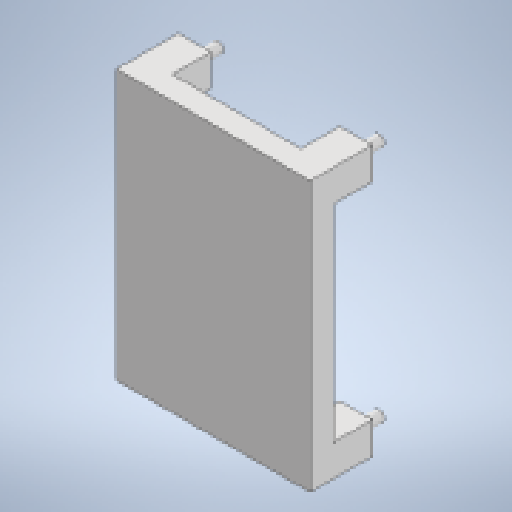
# Autodesk Inventor part: head_box
Saved by Autodesk Inventor 2024 (Build 280153000, 153)
## iProperties
Created: 2024-09-18
Part Number: head_box
Material: 일반
Document SubType Name: Modeling
Designer: Eungang
Density: 1 g/cm^3
Appearance: 기본값
Author: Eungang
Autodesk Inventor part; units mm, degrees
ref_plane "YZ Plane" through (0, 0, 0) normal (1, 0, 0) x (0, 1, 0)
ref_plane "XZ Plane" through (0, 0, 0) normal (0, 1, 0) x (-1, 0, 0)
ref_plane "XY Plane" through (0, 0, 0) normal (0, 0, 1) x (1, 0, 0)
sketch "스케치1" plane through (0, 0, 0) normal (0, 0, 1) x (1, 0, 0)
  circle A0 centre (20.8, -30.8) radius 1.6
  circle A1 centre (20.8, 30.8) radius 1.6
  circle A2 centre (-20.8, -30.8) radius 1.6
  circle A3 centre (-20.8, 30.8) radius 1.6
  line L0 (25, 35) -> (25, -35)
  line L1 (-25, 35) -> (25, 35)
  line L2 (-25, -35) -> (-25, 35)
  line L3 (25, -35) -> (-25, -35)
  line L4 (3.4609, -14.6309) -> (3.4609, -15.4416)
  line L5 (3.4609, -15.4416) -> (-1.9174, -15.4416)
  line L6 (-1.9174, -15.4416) -> (-1.9174, -17.4882)
  line L7 (-1.9174, -17.4882) -> (-2.6391, -17.4882)
  line L8 (-2.6391, -17.4882) -> (-2.6391, -12.5844)
  line L9 (-2.6391, -12.5844) -> (-1.9174, -12.5844)
  line L10 (-1.9174, -12.5844) -> (-1.9174, -14.6309)
  line L11 (-1.9174, -14.6309) -> (3.4609, -14.6309)
  spline S0 degree 3 poles (3.5894, -6.7069) (3.5894, -7.2061) (3.5079, -7.4974) (3.4054, -7.7829) (3.3472, -7.9038) (3.2038, -8.1322) (3.1203, -8.2371) (3.0259, -8.3332) knots 0 0 0 0 0.384557 0.384557 0.692405 0.692405 1 1 1 1
  spline S1 degree 3 poles (3.0259, -8.3332) (2.8735, -8.4928) (2.696, -8.6163) (2.4131, -8.7398) (2.2257, -8.8143) (1.6618, -8.9024) (1.4109, -8.9165) (1.1672, -8.9165) knots 0 0 0 0 0.589252 0.589252 0.824533 0.824533 1 1 1 1
  line L12 (1.1672, -8.9165) -> (-2.6391, -8.9165)
  line L13 (-2.6391, -8.9165) -> (-2.6391, -8.1058)
  line L14 (-2.6391, -8.1058) -> (1.187, -8.1058)
  spline S2 degree 3 poles (1.187, -8.1058) (1.576, -8.1058) (1.7854, -8.0698) (2.0673, -8.0159) (2.2402, -7.948) (2.3981, -7.8438) knots 0 0 0 0 0.340954 0.340954 1 1 1 1
  spline S3 degree 3 poles (2.3981, -7.8438) (2.5057, -7.7728) (2.5951, -7.6834) (2.7648, -7.4325) (2.8129, -7.284) (2.8802, -7.0309) (2.8973, -6.8687) (2.8973, -6.7069) knots 0 0 0 0 0.220643 0.220643 0.518387 0.518387 1 1 1 1
  spline S4 degree 3 poles (2.8973, -6.7069) (2.8973, -6.4866) (2.8694, -6.2573) (2.7554, -5.9796) (2.7065, -5.8804) (2.5606, -5.7003) (2.4845, -5.6319) (2.3981, -5.5749) knots 0 0 0 0 0.605349 0.605349 0.823714 0.823714 1 1 1 1
  spline S5 degree 3 poles (2.3981, -5.5749) (2.2456, -5.4743) (2.0787, -5.4078) (1.787, -5.3484) (1.5677, -5.3129) (1.1672, -5.3129) knots 0 0 0 0 0.613521 0.613521 1 1 1 1
  line L15 (1.1672, -5.3129) -> (-2.6391, -5.3129)
  line L16 (-2.6391, -5.3129) -> (-2.6391, -4.5022)
  line L17 (-2.6391, -4.5022) -> (1.1672, -4.5022)
  spline S6 degree 3 poles (1.1672, -4.5022) (1.7467, -4.5022) (2.0771, -4.578) (2.4094, -4.6758) (2.5476, -4.7346) (2.8054, -4.8878) (2.9214, -4.9794) (3.0259, -5.0855) knots 0 0 0 0 0.39454 0.39454 0.699346 0.699346 1 1 1 1
  spline S7 degree 3 poles (3.0259, -5.0855) (3.188, -5.2476) (3.3119, -5.4359) (3.468, -5.8026) (3.513, -5.9645) (3.576, -6.3201) (3.5894, -6.5148) (3.5894, -6.7069) knots 0 0 0 0 0.387918 0.387918 0.674422 0.674422 1 1 1 1
  line L18 (3.4609, 6.6696) -> (2.838, 6.6696)
  line L19 (2.838, 6.6696) -> (2.838, 7.4457)
  line L20 (2.838, 7.4457) -> (-2.0163, 7.4457)
  line L21 (-2.0163, 7.4457) -> (-2.0163, 6.6696)
  line L22 (-2.0163, 6.6696) -> (-2.6391, 6.6696)
  line L23 (-2.6391, 6.6696) -> (-2.6391, 9.0325)
  line L24 (-2.6391, 9.0325) -> (-2.0163, 9.0325)
  line L25 (-2.0163, 9.0325) -> (-2.0163, 8.2564)
  line L26 (-2.0163, 8.2564) -> (2.838, 8.2564)
  line L27 (2.838, 8.2564) -> (2.838, 9.0325)
  line L28 (2.838, 9.0325) -> (3.4609, 9.0325)
  line L29 (3.4609, 9.0325) -> (3.4609, 6.6696)
  spline S8 degree 3 poles (3.5696, 11.4498) (3.5696, 11.0968) (3.5385, 10.9252) (3.4927, 10.6907) (3.4451, 10.5225) (3.3917, 10.3623) knots 0 0 0 0 0.292547 0.292547 1 1 1 1
  spline S9 degree 3 poles (3.3917, 10.3623) (3.3122, 10.1089) (3.2476, 9.9765) (3.1649, 9.8065) (3.1044, 9.6784) (3.0456, 9.5516) knots 0 0 0 0 0.260501 0.260501 1 1 1 1
  line L30 (3.0456, 9.5516) -> (2.0767, 9.5516)
  line L31 (2.0767, 9.5516) -> (2.0767, 9.6109)
  spline S10 degree 3 poles (2.0767, 9.6109) (2.1724, 9.7066) (2.276, 9.8355) (2.4013, 9.9909) (2.4887, 10.1245) (2.5661, 10.2584) knots 0 0 0 0 0.224538 0.224538 1 1 1 1
  spline S11 degree 3 poles (2.5661, 10.2584) (2.6936, 10.4889) (2.7578, 10.7089) (2.8422, 11.001) (2.8677, 11.2201) (2.8677, 11.4399) knots 0 0 0 0 0.277128 0.277128 1 1 1 1
  spline S12 degree 3 poles (2.8677, 11.4399) (2.8677, 11.6791) (2.8234, 11.9096) (2.6905, 12.2276) (2.6304, 12.347) (2.4562, 12.5833) (2.363, 12.6815) (2.2596, 12.7696) knots 0 0 0 0 0.549193 0.549193 0.79146 0.79146 1 1 1 1
  spline S13 degree 3 poles (2.2596, 12.7696) (2.0598, 12.9378) (1.8287, 13.0612) (1.3654, 13.2321) (1.0093, 13.3332) (0.4158, 13.3332) knots 0 0 0 0 0.528777 0.528777 1 1 1 1
  spline S14 degree 3 poles (0.4158, 13.3332) (-0.1058, 13.3332) (-0.4504, 13.2487) (-0.927, 13.104) (-1.2002, 12.9774) (-1.428, 12.7894) knots 0 0 0 0 0.407318 0.407318 1 1 1 1
  spline S15 degree 3 poles (-1.428, 12.7894) (-1.6106, 12.6333) (-1.7595, 12.4499) (-1.9192, 12.1338) (-1.9723, 12.0047) (-2.0407, 11.7153) (-2.0558, 11.5784) (-2.0558, 11.4399) knots 0 0 0 0 0.529795 0.529795 0.78096 0.78096 1 1 1 1
  spline S16 degree 3 poles (-2.0558, 11.4399) (-2.0558, 11.0983) (-1.9995, 10.8945) (-1.922, 10.6336) (-1.853, 10.4636) (-1.7642, 10.3029) knots 0 0 0 0 0.325292 0.325292 1 1 1 1
  spline S17 degree 3 poles (-1.7642, 10.3029) (-1.6346, 10.0678) (-1.5778, 9.9965) (-1.419, 9.8036) (-1.3331, 9.7017) (-1.255, 9.6158) knots 0 0 0 0 0.538227 0.538227 1 1 1 1
  line L32 (-1.255, 9.6158) -> (-1.255, 9.5516)
  line L33 (-1.255, 9.5516) -> (-2.2338, 9.5516)
  spline S18 degree 3 poles (-2.2338, 9.5516) (-2.3342, 9.7386) (-2.4001, 9.8833) (-2.4926, 10.0908) (-2.5452, 10.2254) (-2.5897, 10.3623) knots 0 0 0 0 0.366727 0.366727 1 1 1 1
  spline S19 degree 3 poles (-2.5897, 10.3623) (-2.6578, 10.586) (-2.6908, 10.783) (-2.7347, 11.0489) (-2.7479, 11.2426) (-2.7479, 11.4349) knots 0 0 0 0 0.286175 0.286175 1 1 1 1
  spline S20 degree 3 poles (-2.7479, 11.4349) (-2.7479, 11.8102) (-2.6884, 12.1794) (-2.4851, 12.6671) (-2.4001, 12.8345) (-2.1695, 13.1574) (-2.0458, 13.2939) (-1.9075, 13.4172) knots 0 0 0 0 0.566594 0.566594 0.797666 0.797666 1 1 1 1
  spline S21 degree 3 poles (-1.9075, 13.4172) (-1.6331, 13.6594) (-1.3194, 13.8381) (-0.7236, 14.0548) (-0.2884, 14.1785) (0.4158, 14.1785) knots 0 0 0 0 0.577352 0.577352 1 1 1 1
  spline S22 degree 3 poles (0.4158, 14.1785) (1.1016, 14.1785) (1.5387, 14.0598) (1.9684, 13.9147) (2.1514, 13.8354) (2.4841, 13.645) (2.6333, 13.5376) (2.7688, 13.4123) knots 0 0 0 0 0.205724 0.205724 0.366116 0.366116 0.515054 0.515054 0.515054 0.515054
  spline S23 degree 3 poles (2.7688, 13.4123) (3.001, 13.2001) (3.1844, 12.9521) (3.4019, 12.4833) (3.465, 12.2871) (3.55, 11.8776) (3.5696, 11.6642) (3.5696, 11.4498) knots 0 0 0 0 0.431078 0.431078 0.708336 0.708336 1 1 1 1
  line L34 (3.4609, 0.9453) -> (0.8063, 3.1154)
  spline S24 degree 3 poles (0.8063, 3.1154) (0.7091, 2.8546) (0.5712, 2.6157) (0.2499, 2.2703) (0.0734, 2.1207) (-0.2854, 1.9573) (-0.4142, 1.9172) (-0.6904, 1.8622) (-0.8369, 1.8499) (-0.9831, 1.8499) knots 0 0 0 0 0.408273 0.408273 0.691747 0.691747 0.83987 0.83987 1 1 1 1
  spline S25 degree 3 poles (-0.9831, 1.8499) (-1.2, 1.8499) (-1.421, 1.8784) (-1.7689, 2.0145) (-1.898, 2.0959) (-2.134, 2.2962) (-2.234, 2.4122) (-2.3178, 2.542) knots 0 0 0 0 0.409869 0.409869 0.705358 0.705358 1 1 1 1
  spline S26 degree 3 poles (-2.3178, 2.542) (-2.4457, 2.7399) (-2.5352, 2.9539) (-2.6309, 3.4845) (-2.6391, 3.7907) (-2.6391, 4.0942) knots 0 0 0 0 0.436998 0.436998 1 1 1 1
  line L35 (-2.6391, 4.0942) -> (-2.6391, 5.6661)
  line L36 (-2.6391, 5.6661) -> (3.4609, 5.6661)
  line L37 (3.4609, 5.6661) -> (3.4609, 4.8554)
  line L38 (3.4609, 4.8554) -> (1.0337, 4.8554)
  line L39 (1.0337, 4.8554) -> (1.0337, 3.9261)
  line L40 (1.0337, 3.9261) -> (3.4609, 1.9982)
  line L41 (3.4609, 1.9982) -> (3.4609, 0.9453)
  spline S27 degree 3 poles (3.5696, -1.9218) (3.5696, -2.2748) (3.5385, -2.4464) (3.4927, -2.6809) (3.4451, -2.849) (3.3917, -3.0093) knots 0 0 0 0 0.292547 0.292547 1 1 1 1
  spline S28 degree 3 poles (3.3917, -3.0093) (3.3122, -3.2627) (3.2476, -3.3951) (3.1649, -3.5651) (3.1044, -3.6932) (3.0456, -3.82) knots 0 0 0 0 0.260501 0.260501 1 1 1 1
  line L42 (3.0456, -3.82) -> (2.0767, -3.82)
  line L43 (2.0767, -3.82) -> (2.0767, -3.7607)
  spline S29 degree 3 poles (2.0767, -3.7607) (2.1724, -3.665) (2.276, -3.5361) (2.4013, -3.3806) (2.4887, -3.2471) (2.5661, -3.1131) knots 0 0 0 0 0.224538 0.224538 1 1 1 1
  spline S30 degree 3 poles (2.5661, -3.1131) (2.6936, -2.8826) (2.7578, -2.6627) (2.8422, -2.3706) (2.8677, -2.1514) (2.8677, -1.9317) knots 0 0 0 0 0.277128 0.277128 1 1 1 1
  spline S31 degree 3 poles (2.8677, -1.9317) (2.8677, -1.6925) (2.8234, -1.462) (2.6905, -1.144) (2.6304, -1.0246) (2.4562, -0.7882) (2.363, -0.6901) (2.2596, -0.6019) knots 0 0 0 0 0.549193 0.549193 0.79146 0.79146 1 1 1 1
  spline S32 degree 3 poles (2.2596, -0.6019) (2.0598, -0.4338) (1.8287, -0.3103) (1.3654, -0.1394) (1.0093, -0.0384) (0.4158, -0.0384) knots 0 0 0 0 0.528777 0.528777 1 1 1 1
  spline S33 degree 3 poles (0.4158, -0.0384) (-0.1058, -0.0384) (-0.4504, -0.1228) (-0.927, -0.2675) (-1.2002, -0.3941) (-1.428, -0.5822) knots 0 0 0 0 0.407318 0.407318 1 1 1 1
  spline S34 degree 3 poles (-1.428, -0.5822) (-1.6106, -0.7383) (-1.7595, -0.9217) (-1.9192, -1.2377) (-1.9723, -1.3669) (-2.0407, -1.6563) (-2.0558, -1.7931) (-2.0558, -1.9317) knots 0 0 0 0 0.529795 0.529795 0.78096 0.78096 1 1 1 1
  spline S35 degree 3 poles (-2.0558, -1.9317) (-2.0558, -2.2732) (-1.9995, -2.4771) (-1.922, -2.7379) (-1.853, -2.908) (-1.7642, -3.0686) knots 0 0 0 0 0.325292 0.325292 1 1 1 1
  spline S36 degree 3 poles (-1.7642, -3.0686) (-1.6346, -3.3037) (-1.5778, -3.3751) (-1.419, -3.568) (-1.3331, -3.6699) (-1.255, -3.7557) knots 0 0 0 0 0.538227 0.538227 1 1 1 1
  line L44 (-1.255, -3.7557) -> (-1.255, -3.82)
  line L45 (-1.255, -3.82) -> (-2.2338, -3.82)
  spline S37 degree 3 poles (-2.2338, -3.82) (-2.3342, -3.6329) (-2.4001, -3.4883) (-2.4926, -3.2807) (-2.5452, -3.1462) (-2.5897, -3.0093) knots 0 0 0 0 0.366727 0.366727 1 1 1 1
  spline S38 degree 3 poles (-2.5897, -3.0093) (-2.6578, -2.7855) (-2.6908, -2.5886) (-2.7347, -2.3227) (-2.7479, -2.129) (-2.7479, -1.9366) knots 0 0 0 0 0.286175 0.286175 1 1 1 1
  spline S39 degree 3 poles (-2.7479, -1.9366) (-2.7479, -1.5613) (-2.6884, -1.1922) (-2.4851, -0.7045) (-2.4001, -0.5371) (-2.1695, -0.2142) (-2.0458, -0.0776) (-1.9075, 0.0456) knots 0 0 0 0 0.566594 0.566594 0.797666 0.797666 1 1 1 1
  spline S40 degree 3 poles (-1.9075, 0.0456) (-1.6331, 0.2878) (-1.3194, 0.4666) (-0.7236, 0.6832) (-0.2884, 0.8069) (0.4158, 0.8069) knots 0 0 0 0 0.577352 0.577352 1 1 1 1
  spline S41 degree 3 poles (0.4158, 0.8069) (1.1016, 0.8069) (1.5387, 0.6882) (1.9684, 0.5432) (2.1514, 0.4638) (2.4841, 0.2734) (2.6333, 0.166) (2.7688, 0.0407) knots 0 0 0 0 0.205724 0.205724 0.366116 0.366116 0.515054 0.515054 0.515054 0.515054
  spline S42 degree 3 poles (2.7688, 0.0407) (3.001, -0.1714) (3.1844, -0.4194) (3.4019, -0.8882) (3.465, -1.0845) (3.55, -1.494) (3.5696, -1.7074) (3.5696, -1.9218) knots 0 0 0 0 0.431078 0.431078 0.708336 0.708336 1 1 1 1
  line L46 (3.4609, -12.2038) -> (2.838, -12.2038)
  line L47 (2.838, -12.2038) -> (2.838, -11.4277)
  line L48 (2.838, -11.4277) -> (-2.0163, -11.4277)
  line L49 (-2.0163, -11.4277) -> (-2.0163, -12.2038)
  line L50 (-2.0163, -12.2038) -> (-2.6391, -12.2038)
  line L51 (-2.6391, -12.2038) -> (-2.6391, -9.8409)
  line L52 (-2.6391, -9.8409) -> (-2.0163, -9.8409)
  line L53 (-2.0163, -9.8409) -> (-2.0163, -10.617)
  line L54 (-2.0163, -10.617) -> (2.838, -10.617)
  line L55 (2.838, -10.617) -> (2.838, -9.8409)
  line L56 (2.838, -9.8409) -> (3.4609, -9.8409)
  line L57 (3.4609, -9.8409) -> (3.4609, -12.2038)
  line L58 (-25, -35) -> (25, -35)
  line L59 (25, -35) -> (25, 35)
  line L60 (25, 35) -> (-25, 35)
  line L61 (-25, 35) -> (-25, -35)
  circle A4 centre (-20.8, 30.8) radius 4.2
  circle A5 centre (-20.8, -30.8) radius 4.2
  circle A6 centre (20.8, -30.8) radius 4.2
  circle A7 centre (20.8, 30.8) radius 4.2
  line L62 (-16.6, 26.6) -> (-25, 26.6)
  line L63 (-25, 26.6) -> (-25, 35)
  line L64 (-25, 35) -> (-16.6, 35)
  line L65 (-16.6, 35) -> (-16.6, 26.6)
  line L66 (-16.6, -26.6) -> (-25, -26.6)
  line L67 (-25, -26.6) -> (-25, -35)
  line L68 (-25, -35) -> (-16.6, -35)
  line L69 (-16.6, -35) -> (-16.6, -26.6)
  line L70 (16.6, -26.6) -> (25, -26.6)
  line L71 (25, -26.6) -> (25, -35)
  line L72 (25, -35) -> (16.6, -35)
  line L73 (16.6, -35) -> (16.6, -26.6)
  line L74 (16.6, 26.6) -> (25, 26.6)
  line L75 (25, 26.6) -> (25, 35)
  line L76 (25, 35) -> (16.6, 35)
  line L77 (16.6, 35) -> (16.6, 26.6)
  point P0 (0, 0)
  point P1 (-16.6, -30.8)
  point P2 (-20.8, -35)
  point P3 (-20.8, -26.6)
  point P4 (-25, -30.8)
  point P5 (16.6, -30.8)
  point P6 (20.8, -35)
  point P7 (20.8, -26.6)
  point P8 (25, -30.8)
  point P9 (-16.6, 30.8)
  point P10 (-20.8, 35)
  point P11 (-20.8, 26.6)
  point P12 (-25, 30.8)
  point P13 (16.6, 30.8)
  point P14 (20.8, 35)
  point P15 (20.8, 26.6)
  point P16 (25, 30.8)
  constraints: 40 end point, 10 parallel, 5 horizontal, 5 perpendicular, 4 centre point, 4 coincident, 4 point on line, 4 tangent
extrude "돌출1" add sketch "스케치1" along normal blind 10 contours A0 | A1 | A2 | A3 | L0 A7 L1 | A7 | L0 L74 A7 | A7 L77 L1 | L74 L77 A7 | L0 A6 L70 | L65 A4 L1 | A6 | L0 L3 A6 | A6 L73 L70 | A4 L2 L1 | A4 | L65 L62 A4 | L3 L73 A6 | A4 L62 L2 | L3 A5 L69 | L66 A5 L2 | L3 L2 A5 | A5 | A5 L66 L69
sketch "스케치2" plane through (-20.8, -30.8, 10) normal (0, 0, 1) x (1, 0, 0)
  circle A0 centre (41.6, 0) radius 1.6
  circle A1 centre (41.6, 61.6) radius 1.6
  circle A2 centre (0, 0) radius 1.6
  circle A3 centre (0, 61.6) radius 1.6
  line L0 (45.8, 65.8) -> (45.8, -4.2)
  line L1 (-4.2, 65.8) -> (45.8, 65.8)
  line L2 (-4.2, -4.2) -> (-4.2, 65.8)
  line L3 (45.8, -4.2) -> (-4.2, -4.2)
  line L4 (24.2609, 16.1691) -> (24.2609, 15.3584)
  line L5 (24.2609, 15.3584) -> (18.8826, 15.3584)
  line L6 (18.8826, 15.3584) -> (18.8826, 13.3118)
  line L7 (18.8826, 13.3118) -> (18.1609, 13.3118)
  line L8 (18.1609, 13.3118) -> (18.1609, 18.2156)
  line L9 (18.1609, 18.2156) -> (18.8826, 18.2156)
  line L10 (18.8826, 18.2156) -> (18.8826, 16.1691)
  line L11 (18.8826, 16.1691) -> (24.2609, 16.1691)
  spline S0 degree 3 poles (24.3894, 24.0931) (24.3894, 23.5939) (24.3079, 23.3026) (24.2054, 23.0171) (24.1472, 22.8962) (24.0038, 22.6678) (23.9203, 22.5629) (23.8259, 22.4668) knots 0 0 0 0 0.384557 0.384557 0.692405 0.692405 1 1 1 1
  spline S1 degree 3 poles (23.8259, 22.4668) (23.6735, 22.3072) (23.496, 22.1837) (23.2131, 22.0602) (23.0257, 21.9857) (22.4618, 21.8976) (22.2109, 21.8835) (21.9672, 21.8835) knots 0 0 0 0 0.589252 0.589252 0.824533 0.824533 1 1 1 1
  line L12 (21.9672, 21.8835) -> (18.1609, 21.8835)
  line L13 (18.1609, 21.8835) -> (18.1609, 22.6942)
  line L14 (18.1609, 22.6942) -> (21.987, 22.6942)
  spline S2 degree 3 poles (21.987, 22.6942) (22.376, 22.6942) (22.5854, 22.7302) (22.8673, 22.7841) (23.0402, 22.852) (23.1981, 22.9562) knots 0 0 0 0 0.340954 0.340954 1 1 1 1
  spline S3 degree 3 poles (23.1981, 22.9562) (23.3057, 23.0272) (23.3951, 23.1166) (23.5648, 23.3675) (23.6129, 23.516) (23.6802, 23.7691) (23.6973, 23.9313) (23.6973, 24.0931) knots 0 0 0 0 0.220643 0.220643 0.518387 0.518387 1 1 1 1
  spline S4 degree 3 poles (23.6973, 24.0931) (23.6973, 24.3134) (23.6694, 24.5427) (23.5554, 24.8204) (23.5065, 24.9196) (23.3606, 25.0997) (23.2845, 25.1681) (23.1981, 25.2251) knots 0 0 0 0 0.605349 0.605349 0.823714 0.823714 1 1 1 1
  spline S5 degree 3 poles (23.1981, 25.2251) (23.0456, 25.3257) (22.8787, 25.3922) (22.587, 25.4516) (22.3677, 25.4871) (21.9672, 25.4871) knots 0 0 0 0 0.613521 0.613521 1 1 1 1
  line L15 (21.9672, 25.4871) -> (18.1609, 25.4871)
  line L16 (18.1609, 25.4871) -> (18.1609, 26.2978)
  line L17 (18.1609, 26.2978) -> (21.9672, 26.2978)
  spline S6 degree 3 poles (21.9672, 26.2978) (22.5467, 26.2978) (22.8771, 26.222) (23.2094, 26.1242) (23.3476, 26.0654) (23.6054, 25.9122) (23.7214, 25.8206) (23.8259, 25.7145) knots 0 0 0 0 0.39454 0.39454 0.699346 0.699346 1 1 1 1
  spline S7 degree 3 poles (23.8259, 25.7145) (23.988, 25.5524) (24.1119, 25.3641) (24.268, 24.9974) (24.313, 24.8355) (24.376, 24.4799) (24.3894, 24.2852) (24.3894, 24.0931) knots 0 0 0 0 0.387918 0.387918 0.674422 0.674422 1 1 1 1
  line L18 (24.2609, 37.4696) -> (23.638, 37.4696)
  line L19 (23.638, 37.4696) -> (23.638, 38.2457)
  line L20 (23.638, 38.2457) -> (18.7837, 38.2457)
  line L21 (18.7837, 38.2457) -> (18.7837, 37.4696)
  line L22 (18.7837, 37.4696) -> (18.1609, 37.4696)
  line L23 (18.1609, 37.4696) -> (18.1609, 39.8325)
  line L24 (18.1609, 39.8325) -> (18.7837, 39.8325)
  line L25 (18.7837, 39.8325) -> (18.7837, 39.0564)
  line L26 (18.7837, 39.0564) -> (23.638, 39.0564)
  line L27 (23.638, 39.0564) -> (23.638, 39.8325)
  line L28 (23.638, 39.8325) -> (24.2609, 39.8325)
  line L29 (24.2609, 39.8325) -> (24.2609, 37.4696)
  spline S8 degree 3 poles (24.3696, 42.2498) (24.3696, 41.8968) (24.3385, 41.7252) (24.2927, 41.4907) (24.2451, 41.3225) (24.1917, 41.1623) knots 0 0 0 0 0.292547 0.292547 1 1 1 1
  spline S9 degree 3 poles (24.1917, 41.1623) (24.1122, 40.9089) (24.0476, 40.7765) (23.9649, 40.6065) (23.9044, 40.4784) (23.8456, 40.3516) knots 0 0 0 0 0.260501 0.260501 1 1 1 1
  line L30 (23.8456, 40.3516) -> (22.8767, 40.3516)
  line L31 (22.8767, 40.3516) -> (22.8767, 40.4109)
  spline S10 degree 3 poles (22.8767, 40.4109) (22.9724, 40.5066) (23.076, 40.6355) (23.2013, 40.7909) (23.2887, 40.9245) (23.3661, 41.0584) knots 0 0 0 0 0.224538 0.224538 1 1 1 1
  spline S11 degree 3 poles (23.3661, 41.0584) (23.4936, 41.2889) (23.5578, 41.5089) (23.6422, 41.801) (23.6677, 42.0201) (23.6677, 42.2399) knots 0 0 0 0 0.277128 0.277128 1 1 1 1
  spline S12 degree 3 poles (23.6677, 42.2399) (23.6677, 42.4791) (23.6234, 42.7096) (23.4905, 43.0276) (23.4304, 43.147) (23.2562, 43.3833) (23.163, 43.4815) (23.0596, 43.5696) knots 0 0 0 0 0.549193 0.549193 0.79146 0.79146 1 1 1 1
  spline S13 degree 3 poles (23.0596, 43.5696) (22.8598, 43.7378) (22.6287, 43.8612) (22.1654, 44.0321) (21.8093, 44.1332) (21.2158, 44.1332) knots 0 0 0 0 0.528777 0.528777 1 1 1 1
  spline S14 degree 3 poles (21.2158, 44.1332) (20.6942, 44.1332) (20.3496, 44.0487) (19.873, 43.904) (19.5998, 43.7774) (19.372, 43.5894) knots 0 0 0 0 0.407318 0.407318 1 1 1 1
  spline S15 degree 3 poles (19.372, 43.5894) (19.1894, 43.4333) (19.0405, 43.2499) (18.8808, 42.9338) (18.8277, 42.8047) (18.7593, 42.5153) (18.7442, 42.3784) (18.7442, 42.2399) knots 0 0 0 0 0.529795 0.529795 0.78096 0.78096 1 1 1 1
  spline S16 degree 3 poles (18.7442, 42.2399) (18.7442, 41.8983) (18.8005, 41.6945) (18.878, 41.4336) (18.947, 41.2636) (19.0358, 41.1029) knots 0 0 0 0 0.325292 0.325292 1 1 1 1
  spline S17 degree 3 poles (19.0358, 41.1029) (19.1654, 40.8678) (19.2222, 40.7965) (19.381, 40.6036) (19.4669, 40.5017) (19.545, 40.4158) knots 0 0 0 0 0.538227 0.538227 1 1 1 1
  line L32 (19.545, 40.4158) -> (19.545, 40.3516)
  line L33 (19.545, 40.3516) -> (18.5662, 40.3516)
  spline S18 degree 3 poles (18.5662, 40.3516) (18.4658, 40.5386) (18.3999, 40.6833) (18.3074, 40.8908) (18.2548, 41.0254) (18.2103, 41.1623) knots 0 0 0 0 0.366727 0.366727 1 1 1 1
  spline S19 degree 3 poles (18.2103, 41.1623) (18.1422, 41.386) (18.1092, 41.583) (18.0653, 41.8489) (18.0521, 42.0426) (18.0521, 42.2349) knots 0 0 0 0 0.286175 0.286175 1 1 1 1
  spline S20 degree 3 poles (18.0521, 42.2349) (18.0521, 42.6102) (18.1116, 42.9794) (18.3149, 43.4671) (18.3999, 43.6345) (18.6305, 43.9574) (18.7542, 44.0939) (18.8925, 44.2172) knots 0 0 0 0 0.566594 0.566594 0.797666 0.797666 1 1 1 1
  spline S21 degree 3 poles (18.8925, 44.2172) (19.1669, 44.4594) (19.4806, 44.6381) (20.0764, 44.8548) (20.5116, 44.9785) (21.2158, 44.9785) knots 0 0 0 0 0.577352 0.577352 1 1 1 1
  spline S22 degree 3 poles (21.2158, 44.9785) (21.9016, 44.9785) (22.3387, 44.8598) (22.7684, 44.7147) (22.9514, 44.6354) (23.2841, 44.445) (23.4333, 44.3376) (23.5688, 44.2123) knots 0 0 0 0 0.205724 0.205724 0.366116 0.366116 0.515054 0.515054 0.515054 0.515054
  spline S23 degree 3 poles (23.5688, 44.2123) (23.801, 44.0001) (23.9844, 43.7521) (24.2019, 43.2833) (24.265, 43.0871) (24.35, 42.6776) (24.3696, 42.4642) (24.3696, 42.2498) knots 0 0 0 0 0.431078 0.431078 0.708336 0.708336 1 1 1 1
  line L34 (24.2609, 31.7453) -> (21.6063, 33.9154)
  spline S24 degree 3 poles (21.6063, 33.9154) (21.5091, 33.6546) (21.3712, 33.4157) (21.0499, 33.0703) (20.8734, 32.9207) (20.5146, 32.7573) (20.3858, 32.7172) (20.1096, 32.6622) (19.9631, 32.6499) (19.8169, 32.6499) knots 0 0 0 0 0.408273 0.408273 0.691747 0.691747 0.83987 0.83987 1 1 1 1
  spline S25 degree 3 poles (19.8169, 32.6499) (19.6, 32.6499) (19.379, 32.6784) (19.0311, 32.8145) (18.902, 32.8959) (18.666, 33.0962) (18.566, 33.2122) (18.4822, 33.342) knots 0 0 0 0 0.409869 0.409869 0.705358 0.705358 1 1 1 1
  spline S26 degree 3 poles (18.4822, 33.342) (18.3543, 33.5399) (18.2648, 33.7539) (18.1691, 34.2845) (18.1609, 34.5907) (18.1609, 34.8942) knots 0 0 0 0 0.436998 0.436998 1 1 1 1
  line L35 (18.1609, 34.8942) -> (18.1609, 36.4661)
  line L36 (18.1609, 36.4661) -> (24.2609, 36.4661)
  line L37 (24.2609, 36.4661) -> (24.2609, 35.6554)
  line L38 (24.2609, 35.6554) -> (21.8337, 35.6554)
  line L39 (21.8337, 35.6554) -> (21.8337, 34.7261)
  line L40 (21.8337, 34.7261) -> (24.2609, 32.7982)
  line L41 (24.2609, 32.7982) -> (24.2609, 31.7453)
  spline S27 degree 3 poles (24.3696, 28.8782) (24.3696, 28.5252) (24.3385, 28.3536) (24.2927, 28.1191) (24.2451, 27.951) (24.1917, 27.7907) knots 0 0 0 0 0.292547 0.292547 1 1 1 1
  spline S28 degree 3 poles (24.1917, 27.7907) (24.1122, 27.5373) (24.0476, 27.4049) (23.9649, 27.2349) (23.9044, 27.1068) (23.8456, 26.98) knots 0 0 0 0 0.260501 0.260501 1 1 1 1
  line L42 (23.8456, 26.98) -> (22.8767, 26.98)
  line L43 (22.8767, 26.98) -> (22.8767, 27.0393)
  spline S29 degree 3 poles (22.8767, 27.0393) (22.9724, 27.135) (23.076, 27.2639) (23.2013, 27.4194) (23.2887, 27.5529) (23.3661, 27.6869) knots 0 0 0 0 0.224538 0.224538 1 1 1 1
  spline S30 degree 3 poles (23.3661, 27.6869) (23.4936, 27.9174) (23.5578, 28.1373) (23.6422, 28.4294) (23.6677, 28.6486) (23.6677, 28.8683) knots 0 0 0 0 0.277128 0.277128 1 1 1 1
  spline S31 degree 3 poles (23.6677, 28.8683) (23.6677, 29.1075) (23.6234, 29.338) (23.4905, 29.656) (23.4304, 29.7754) (23.2562, 30.0118) (23.163, 30.1099) (23.0596, 30.1981) knots 0 0 0 0 0.549193 0.549193 0.79146 0.79146 1 1 1 1
  spline S32 degree 3 poles (23.0596, 30.1981) (22.8598, 30.3662) (22.6287, 30.4897) (22.1654, 30.6606) (21.8093, 30.7616) (21.2158, 30.7616) knots 0 0 0 0 0.528777 0.528777 1 1 1 1
  spline S33 degree 3 poles (21.2158, 30.7616) (20.6942, 30.7616) (20.3496, 30.6772) (19.873, 30.5325) (19.5998, 30.4059) (19.372, 30.2178) knots 0 0 0 0 0.407318 0.407318 1 1 1 1
  spline S34 degree 3 poles (19.372, 30.2178) (19.1894, 30.0617) (19.0405, 29.8783) (18.8808, 29.5623) (18.8277, 29.4331) (18.7593, 29.1437) (18.7442, 29.0069) (18.7442, 28.8683) knots 0 0 0 0 0.529795 0.529795 0.78096 0.78096 1 1 1 1
  spline S35 degree 3 poles (18.7442, 28.8683) (18.7442, 28.5268) (18.8005, 28.3229) (18.878, 28.0621) (18.947, 27.892) (19.0358, 27.7314) knots 0 0 0 0 0.325292 0.325292 1 1 1 1
  spline S36 degree 3 poles (19.0358, 27.7314) (19.1654, 27.4963) (19.2222, 27.4249) (19.381, 27.232) (19.4669, 27.1301) (19.545, 27.0443) knots 0 0 0 0 0.538227 0.538227 1 1 1 1
  line L44 (19.545, 27.0443) -> (19.545, 26.98)
  line L45 (19.545, 26.98) -> (18.5662, 26.98)
  spline S37 degree 3 poles (18.5662, 26.98) (18.4658, 27.1671) (18.3999, 27.3117) (18.3074, 27.5193) (18.2548, 27.6538) (18.2103, 27.7907) knots 0 0 0 0 0.366727 0.366727 1 1 1 1
  spline S38 degree 3 poles (18.2103, 27.7907) (18.1422, 28.0145) (18.1092, 28.2114) (18.0653, 28.4773) (18.0521, 28.671) (18.0521, 28.8634) knots 0 0 0 0 0.286175 0.286175 1 1 1 1
  spline S39 degree 3 poles (18.0521, 28.8634) (18.0521, 29.2387) (18.1116, 29.6078) (18.3149, 30.0955) (18.3999, 30.2629) (18.6305, 30.5858) (18.7542, 30.7224) (18.8925, 30.8456) knots 0 0 0 0 0.566594 0.566594 0.797666 0.797666 1 1 1 1
  spline S40 degree 3 poles (18.8925, 30.8456) (19.1669, 31.0878) (19.4806, 31.2666) (20.0764, 31.4832) (20.5116, 31.6069) (21.2158, 31.6069) knots 0 0 0 0 0.577352 0.577352 1 1 1 1
  spline S41 degree 3 poles (21.2158, 31.6069) (21.9016, 31.6069) (22.3387, 31.4882) (22.7684, 31.3432) (22.9514, 31.2638) (23.2841, 31.0734) (23.4333, 30.966) (23.5688, 30.8407) knots 0 0 0 0 0.205724 0.205724 0.366116 0.366116 0.515054 0.515054 0.515054 0.515054
  spline S42 degree 3 poles (23.5688, 30.8407) (23.801, 30.6286) (23.9844, 30.3806) (24.2019, 29.9118) (24.265, 29.7155) (24.35, 29.306) (24.3696, 29.0926) (24.3696, 28.8782) knots 0 0 0 0 0.431078 0.431078 0.708336 0.708336 1 1 1 1
  line L46 (24.2609, 18.5962) -> (23.638, 18.5962)
  line L47 (23.638, 18.5962) -> (23.638, 19.3723)
  line L48 (23.638, 19.3723) -> (18.7837, 19.3723)
  line L49 (18.7837, 19.3723) -> (18.7837, 18.5962)
  line L50 (18.7837, 18.5962) -> (18.1609, 18.5962)
  line L51 (18.1609, 18.5962) -> (18.1609, 20.9591)
  line L52 (18.1609, 20.9591) -> (18.7837, 20.9591)
  line L53 (18.7837, 20.9591) -> (18.7837, 20.183)
  line L54 (18.7837, 20.183) -> (23.638, 20.183)
  line L55 (23.638, 20.183) -> (23.638, 20.9591)
  line L56 (23.638, 20.9591) -> (24.2609, 20.9591)
  line L57 (24.2609, 20.9591) -> (24.2609, 18.5962)
  point P0 (20.8, 30.8)
extrude "돌출2" add sketch "스케치2" along normal blind 6 contours A0 | A1 | A2 | A3 | L0 L3 L2 L1 | L4 L5 L6 L7 L8 L9 L10 L11 | S0 S1 L12 L13 L14 S2 S3 S4 S5 L15 L16 L17 S6 S7 | L18 L19 L20 L21 L22 L23 L24 L25 L26 L27 L28 L29 | S8 S9 L30 L31 S10 S11 S12 S13 S14 S15 S16 S17 L32 L33 S18 S19 S20 S21 S22 S23 | L34 S24 S25 S26 L35 L36 L37 L38 L39 L40 L41 | S27 S28 L42 L43 S29 S30 S31 S32 S33 S34 S35 S36 L44 L45 S37 S38 S39 S40 S41 S42 | L46 L47 L48 L49 L50 L51 L52 L53 L54 L55 L56 L57
sketch "스케치4" plane through (20.8, -30.8, 0) normal (0, 0, -1) x (-1, 0, 0)
  circle A0 centre (0, 0) radius 1.6 projected
  circle A1 centre (0, 61.6) radius 1.6 projected
  circle A2 centre (41.6, 0) radius 1.6 projected
  circle A3 centre (41.6, 61.6) radius 1.6 projected
  line L0 (-4.2, 65.8) -> (-4.2, -4.2) projected
  line L1 (-4.2, -4.2) -> (45.8, -4.2) projected
  line L2 (45.8, -4.2) -> (45.8, 65.8) projected
  line L3 (45.8, 65.8) -> (-4.2, 65.8) projected
  line L4 (17.3391, 15.3584) -> (17.3391, 16.1691) projected
  line L5 (17.3391, 16.1691) -> (22.7174, 16.1691) projected
  line L6 (22.7174, 16.1691) -> (22.7174, 18.2156) projected
  line L7 (22.7174, 18.2156) -> (23.4391, 18.2156) projected
  line L8 (23.4391, 18.2156) -> (23.4391, 13.3118) projected
  line L9 (23.4391, 13.3118) -> (22.7174, 13.3118) projected
  line L10 (22.7174, 13.3118) -> (22.7174, 15.3584) projected
  line L11 (22.7174, 15.3584) -> (17.3391, 15.3584) projected
  spline S0 degree 2 poles (17.7741, 22.4668) (17.4874, 22.7584) (17.2106, 23.5296) (17.2106, 24.0931) knots 0 0 0 1 2 2 2 projected
  spline S1 degree 2 poles (17.2106, 24.0931) (17.2106, 24.6319) (17.4924, 25.4328) (17.7741, 25.7145) knots 0 0 0 1 2 2 2 projected
  spline S2 degree 2 poles (17.7741, 25.7145) (18.0905, 26.0358) (18.9803, 26.2978) (19.6328, 26.2978) knots 0 0 0 1 2 2 2 projected
  line L12 (19.6328, 26.2978) -> (23.4391, 26.2978) projected
  line L13 (23.4391, 26.2978) -> (23.4391, 25.4871) projected
  line L14 (23.4391, 25.4871) -> (19.6328, 25.4871) projected
  spline S3 degree 2 poles (19.6328, 25.4871) (19.2077, 25.4871) (18.6343, 25.3784) (18.4019, 25.2251) knots 0 0 0 1 2 2 2 projected
  spline S4 degree 2 poles (18.4019, 25.2251) (18.1548, 25.062) (17.9027, 24.4985) (17.9027, 24.0931) knots 0 0 0 1 2 2 2 projected
  spline S5 degree 2 poles (17.9027, 24.0931) (17.9027, 23.7125) (18.1548, 23.1193) (18.4019, 22.9562) knots 0 0 0 1 2 2 2 projected
  spline S6 degree 2 poles (18.4019, 22.9562) (18.6343, 22.8029) (19.2028, 22.6942) (19.613, 22.6942) knots 0 0 0 1 2 2 2 projected
  line L15 (19.613, 22.6942) -> (23.4391, 22.6942) projected
  line L16 (23.4391, 22.6942) -> (23.4391, 21.8835) projected
  line L17 (23.4391, 21.8835) -> (19.6328, 21.8835) projected
  spline S7 degree 2 poles (19.6328, 21.8835) (18.9951, 21.8835) (18.0856, 22.1405) (17.7741, 22.4668) knots 0 0 0 1 2 2 2 projected
  line L18 (17.962, 37.4696) -> (17.3391, 37.4696) projected
  line L19 (17.3391, 37.4696) -> (17.3391, 39.8325) projected
  line L20 (17.3391, 39.8325) -> (17.962, 39.8325) projected
  line L21 (17.962, 39.8325) -> (17.962, 39.0564) projected
  line L22 (17.962, 39.0564) -> (22.8163, 39.0564) projected
  line L23 (22.8163, 39.0564) -> (22.8163, 39.8325) projected
  line L24 (22.8163, 39.8325) -> (23.4391, 39.8325) projected
  line L25 (23.4391, 39.8325) -> (23.4391, 37.4696) projected
  line L26 (23.4391, 37.4696) -> (22.8163, 37.4696) projected
  line L27 (22.8163, 37.4696) -> (22.8163, 38.2457) projected
  line L28 (22.8163, 38.2457) -> (17.962, 38.2457) projected
  line L29 (17.962, 38.2457) -> (17.962, 37.4696) projected
  spline S8 degree 2 poles (17.4083, 41.1623) (17.3194, 41.4292) (17.2304, 41.884) (17.2304, 42.2498) knots 0 0 0 1 2 2 2 projected
  spline S9 degree 2 poles (17.2304, 42.2498) (17.2304, 42.843) (17.6308, 43.8464) (18.0312, 44.2123) knots 0 0 0 1 2 2 2 projected
  spline S10 degree 2 poles (18.0312, 44.2123) (18.4267, 44.5781) (19.613, 44.9785) (20.3842, 44.9785) knots 0 0 0 1 2 2 2 projected
  spline S11 degree 2 poles (20.3842, 44.9785) (21.1504, 44.9785) (22.2874, 44.5879) (22.7075, 44.2172) knots 0 0 0 1 2 2 2 projected
  spline S12 degree 2 poles (22.7075, 44.2172) (23.1178, 43.8514) (23.5479, 42.8529) (23.5479, 42.2349) knots 0 0 0 1 2 2 2 projected
  spline S13 degree 2 poles (23.5479, 42.2349) (23.5479, 41.9285) (23.4589, 41.3896) (23.3897, 41.1623) knots 0 0 0 1 2 2 2 projected
  spline S14 degree 2 poles (23.3897, 41.1623) (23.3254, 40.9645) (23.1425, 40.5542) (23.0338, 40.3516) knots 0 0 0 1 2 2 2 projected
  line L30 (23.0338, 40.3516) -> (22.055, 40.3516) projected
  line L31 (22.055, 40.3516) -> (22.055, 40.4158) projected
  spline S15 degree 2 poles (22.055, 40.4158) (22.1539, 40.5246) (22.4307, 40.8607) (22.5642, 41.1029) knots 0 0 0 1 2 2 2 projected
  spline S16 degree 2 poles (22.5642, 41.1029) (22.6927, 41.3353) (22.8558, 41.884) (22.8558, 42.2399) knots 0 0 0 1 2 2 2 projected
  spline S17 degree 2 poles (22.8558, 42.2399) (22.8558, 42.6304) (22.5345, 43.3274) (22.228, 43.5894) knots 0 0 0 1 2 2 2 projected
  spline S18 degree 2 poles (22.228, 43.5894) (21.9166, 43.8464) (20.9724, 44.1332) (20.3842, 44.1332) knots 0 0 0 1 2 2 2 projected
  spline S19 degree 2 poles (20.3842, 44.1332) (19.7564, 44.1332) (18.8518, 43.8316) (18.5404, 43.5696) knots 0 0 0 1 2 2 2 projected
  spline S20 degree 2 poles (18.5404, 43.5696) (18.2388, 43.3126) (17.9323, 42.6255) (17.9323, 42.2399) knots 0 0 0 1 2 2 2 projected
  spline S21 degree 2 poles (17.9323, 42.2399) (17.9323, 41.8889) (18.1053, 41.2908) (18.2339, 41.0584) knots 0 0 0 1 2 2 2 projected
  spline S22 degree 2 poles (18.2339, 41.0584) (18.3624, 40.836) (18.6293, 40.5048) (18.7233, 40.4109) knots 0 0 0 1 2 2 2 projected
  line L32 (18.7233, 40.4109) -> (18.7233, 40.3516) projected
  line L33 (18.7233, 40.3516) -> (17.7544, 40.3516) projected
  spline S23 degree 2 poles (17.7544, 40.3516) (17.6604, 40.5542) (17.4874, 40.9101) (17.4083, 41.1623) knots 0 0 0 1 2 2 2 projected
  line L34 (19.9937, 33.9154) -> (17.3391, 31.7453) projected
  line L35 (17.3391, 31.7453) -> (17.3391, 32.7982) projected
  line L36 (17.3391, 32.7982) -> (19.7663, 34.7261) projected
  line L37 (19.7663, 34.7261) -> (19.7663, 35.6554) projected
  line L38 (19.7663, 35.6554) -> (17.3391, 35.6554) projected
  line L39 (17.3391, 35.6554) -> (17.3391, 36.4661) projected
  line L40 (17.3391, 36.4661) -> (23.4391, 36.4661) projected
  line L41 (23.4391, 36.4661) -> (23.4391, 34.8942) projected
  spline S24 degree 2 poles (23.4391, 34.8942) (23.4391, 34.3702) (23.3254, 33.6633) (23.1178, 33.342) knots 0 0 0 1 2 2 2 projected
  spline S25 degree 2 poles (23.1178, 33.342) (22.9102, 33.0207) (22.2626, 32.6499) (21.7831, 32.6499) knots 0 0 0 1 2 2 2 projected
  spline S26 degree 2 poles (21.7831, 32.6499) (21.1158, 32.6499) (20.2112, 33.3321) (19.9937, 33.9154) knots 0 0 0 1 2 2 2 projected
  spline S27 degree 2 poles (17.4083, 27.7907) (17.3194, 28.0576) (17.2304, 28.5124) (17.2304, 28.8782) knots 0 0 0 1 2 2 2 projected
  spline S28 degree 2 poles (17.2304, 28.8782) (17.2304, 29.4714) (17.6308, 30.4749) (18.0312, 30.8407) knots 0 0 0 1 2 2 2 projected
  spline S29 degree 2 poles (18.0312, 30.8407) (18.4267, 31.2065) (19.613, 31.6069) (20.3842, 31.6069) knots 0 0 0 1 2 2 2 projected
  spline S30 degree 2 poles (20.3842, 31.6069) (21.1504, 31.6069) (22.2874, 31.2164) (22.7075, 30.8456) knots 0 0 0 1 2 2 2 projected
  spline S31 degree 2 poles (22.7075, 30.8456) (23.1178, 30.4798) (23.5479, 29.4813) (23.5479, 28.8634) knots 0 0 0 1 2 2 2 projected
  spline S32 degree 2 poles (23.5479, 28.8634) (23.5479, 28.5569) (23.4589, 28.0181) (23.3897, 27.7907) knots 0 0 0 1 2 2 2 projected
  spline S33 degree 2 poles (23.3897, 27.7907) (23.3254, 27.593) (23.1425, 27.1827) (23.0338, 26.98) knots 0 0 0 1 2 2 2 projected
  line L42 (23.0338, 26.98) -> (22.055, 26.98) projected
  line L43 (22.055, 26.98) -> (22.055, 27.0443) projected
  spline S34 degree 2 poles (22.055, 27.0443) (22.1539, 27.153) (22.4307, 27.4892) (22.5642, 27.7314) knots 0 0 0 1 2 2 2 projected
  spline S35 degree 2 poles (22.5642, 27.7314) (22.6927, 27.9637) (22.8558, 28.5124) (22.8558, 28.8683) knots 0 0 0 1 2 2 2 projected
  spline S36 degree 2 poles (22.8558, 28.8683) (22.8558, 29.2588) (22.5345, 29.9558) (22.228, 30.2178) knots 0 0 0 1 2 2 2 projected
  spline S37 degree 2 poles (22.228, 30.2178) (21.9166, 30.4749) (20.9724, 30.7616) (20.3842, 30.7616) knots 0 0 0 1 2 2 2 projected
  spline S38 degree 2 poles (20.3842, 30.7616) (19.7564, 30.7616) (18.8518, 30.4601) (18.5404, 30.1981) knots 0 0 0 1 2 2 2 projected
  spline S39 degree 2 poles (18.5404, 30.1981) (18.2388, 29.941) (17.9323, 29.2539) (17.9323, 28.8683) knots 0 0 0 1 2 2 2 projected
  spline S40 degree 2 poles (17.9323, 28.8683) (17.9323, 28.5174) (18.1053, 27.9192) (18.2339, 27.6869) knots 0 0 0 1 2 2 2 projected
  spline S41 degree 2 poles (18.2339, 27.6869) (18.3624, 27.4644) (18.6293, 27.1332) (18.7233, 27.0393) knots 0 0 0 1 2 2 2 projected
  line L44 (18.7233, 27.0393) -> (18.7233, 26.98) projected
  line L45 (18.7233, 26.98) -> (17.7544, 26.98) projected
  spline S42 degree 2 poles (17.7544, 26.98) (17.6604, 27.1827) (17.4874, 27.5386) (17.4083, 27.7907) knots 0 0 0 1 2 2 2 projected
  line L46 (17.962, 18.5962) -> (17.3391, 18.5962) projected
  line L47 (17.3391, 18.5962) -> (17.3391, 20.9591) projected
  line L48 (17.3391, 20.9591) -> (17.962, 20.9591) projected
  line L49 (17.962, 20.9591) -> (17.962, 20.183) projected
  line L50 (17.962, 20.183) -> (22.8163, 20.183) projected
  line L51 (22.8163, 20.183) -> (22.8163, 20.9591) projected
  line L52 (22.8163, 20.9591) -> (23.4391, 20.9591) projected
  line L53 (23.4391, 20.9591) -> (23.4391, 18.5962) projected
  line L54 (23.4391, 18.5962) -> (22.8163, 18.5962) projected
  line L55 (22.8163, 18.5962) -> (22.8163, 19.3723) projected
  line L56 (22.8163, 19.3723) -> (17.962, 19.3723) projected
  line L57 (17.962, 19.3723) -> (17.962, 18.5962) projected
  circle A4 centre (41.6, 0) radius 1.4
  circle A5 centre (0, 0) radius 1.4
  circle A6 centre (0, 61.6) radius 1.4
  circle A7 centre (41.6, 61.6) radius 1.4
  point P0 (20.8, 30.8)
  dimension "d6" = 0.2
  dimension "d7" = 0.2
  dimension "d8" = 0.2
  dimension "d9" = 0.2
  constraints: 4 centre point
  measures "d6" radial gap between concentric circles of A2 A4
  measures "d7" radial gap between concentric circles of A0 A5
  measures "d8" radial gap between concentric circles of A1 A6
  measures "d9" radial gap between concentric circles of A3 A7
extrude "돌출4" add sketch "스케치4" along normal blind 6 contours A4 | A5 | A6 | A7
thicken "두껍게 하기1" operation cut thickness 0.2 both sides no extend neighbours no toward (0, 1, 0) faces at (5.5333, -35, 14)
thicken "두껍게 하기2" operation cut thickness 0.2 both sides no extend neighbours no toward (0, -1, 0) faces at (-5.5333, 35, 14)
thicken "두껍게 하기3" operation cut thickness 0.2 both sides no extend neighbours no toward (0, -1, 0) faces at (-5.5333, 34.8, 14)
